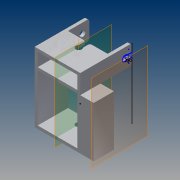
# Autodesk Inventor part: Box
Saved by Autodesk Inventor 2015 SP1 (Build 190203100, 203)
## iProperties
Created: 2015-04-28
Part Number: Box
Material: ABS Plastic
Document SubType Name: Modeling
Designer: Trevor
Density: 1.06 g/cm^3
Appearance: Smooth - White
Author: Trevor
Autodesk Inventor part; units mm, degrees
ref_plane "YZ Plane" through (0, 0, 0) normal (1, 0, 0) x (0, 1, 0)
ref_plane "XZ Plane" through (0, 0, 0) normal (0, 1, 0) x (-1, 0, 0)
ref_plane "XY Plane" through (0, 0, 0) normal (0, 0, 1) x (1, 0, 0)
sketch "Sketch1" plane through (0, 0, 0) normal (0, 0, 1) x (1, 0, 0)
  line L0 (-136.0917, 57.7981) -> (-136.0917, 38.4916) projected
  line L1 (-204.3542, 87.8916) -> (-204.3542, 49.7916) projected
  line L2 (-131.3292, 42.3074) -> (-204.3542, 42.3074)
  line L3 (-204.3542, 42.3074) -> (-204.3542, -69.3801)
  line L4 (-204.3542, -69.3801) -> (-131.3292, -69.3801)
  line L5 (-131.3292, -69.3801) -> (-131.3292, 42.3074)
  line L6 (-131.3292, 43.3824) -> (-131.3292, 52.9074) projected
  line L7 (-204.3542, 87.8916) -> (-204.3542, 49.7916) projected
  line L8 (-165.4906, 16.3449) -> (-168.0727, 16.3449)
  line L9 (-170.1927, 37.5449) -> (-167.6106, 37.5449)
  line L10 (-163.0792, 42.3074) -> (-172.6042, 42.3074) projected
  point P0 (0, 0)
  dimension "d1" = 4.7625
  dimension "d2" = 85.725
  dimension "d30" = 21.2
  constraints: 12 end point, 3 collinear, 2 parallel, 1 horizontal, 1 perpendicular
  measures "d1" distance between parallel lines of L2 L9
  measures "d2" distance between parallel lines of L4 L8
  measures "d30" distance between parallel lines of L8 L9
extrude "Extrusion1" add sketch "Sketch1" against normal blind 82.55
shell "Shell1" thickness 4.7625 removed faces 2 at (-180.0125, 5.0782, -82.55) at (-180.0125, 5.0782, 0)
sketch "Sketch2" plane through (0, 0, -82.55) normal (0, 0, -1) x (-1, 0, 0)
  line L0 (170.1927, 16.3449) -> (167.6106, 16.3449) projected
  line L1 (164.4741, 11.5824) -> (171.2093, 11.5824) projected
  line L2 (199.5917, 37.5449) -> (199.5917, -64.6176) projected
  line L3 (136.0917, -64.6176) -> (136.0917, 37.5449) projected
  line L4 (199.5917, -64.6176) -> (199.5917, 37.5449) projected
  line L5 (199.5917, 11.5824) -> (136.0917, 11.5824)
  line L6 (136.0917, 11.5824) -> (136.0917, 16.3449)
  line L7 (136.0917, 16.3449) -> (199.5917, 16.3449)
  line L8 (199.5917, 16.3449) -> (199.5917, 11.5824)
  point P0 (0, 0)
  constraints: 8 end point, 2 collinear, 2 parallel, 2 point on line, 1 horizontal, 1 perpendicular
extrude "Extrusion2" add sketch "Sketch2" against normal up to surface (82.55 mm away)
sketch "Sketch3" plane through (-204.3542, 42.3074, 0) normal (0, 1, 0) x (1, 0, 0)
  line L0 (73.025, 82.55) -> (0, 82.55) projected
  line L1 (36.5125, 82.55) -> (36.5125, 0)
  line L2 (0, 0) -> (73.025, 0) projected
  arc A0 (33.1449, 30.6087) -> (40.6772, 36.2864) centre (36.5125, 33.9763) ccw
  line L3 (73.025, 0) -> (0, 0) projected
  line L4 (33.1449, 30.6087) -> (39.8801, 30.6087)
  line L5 (39.8801, 30.6087) -> (39.8801, 37.3439)
  line L6 (39.8801, 37.3439) -> (33.1449, 37.3439)
  line L7 (33.1449, 37.3439) -> (33.1449, 30.6087)
  line L8 (33.1449, 30.6087) -> (39.8801, 37.3439) construction
  line L9 (39.8801, 30.6087) -> (33.1449, 37.3439) construction
  line L10 (39.8801, 37.3439) -> (39.8801, 39.3666)
  line L11 (33.1449, 37.3439) -> (33.1449, 39.3666)
  arc A1 (39.8801, 39.3666) -> (40.6772, 36.2864) centre (46.2301, 39.3666) ccw
  arc A2 (32.3478, 36.2864) -> (33.1449, 39.3666) centre (26.7949, 39.3666) ccw
  line L12 (68.2625, 82.55) -> (68.2625, 0) projected
  line L13 (4.7625, 0) -> (4.7625, 82.55) projected
  line L14 (4.7625, 82.55) -> (68.2625, 82.55)
  line L15 (68.2625, 82.55) -> (68.2625, 48.5832)
  line L16 (68.2625, 48.5832) -> (4.7625, 48.5832)
  line L17 (4.7625, 48.5832) -> (4.7625, 82.55)
  line L18 (33.1449, 39.3666) -> (33.1449, 82.55)
  arc A3 (32.3478, 36.2864) -> (33.1449, 30.6087) centre (36.5125, 33.9763) ccw
  line L19 (39.8801, 39.3666) -> (39.8801, 82.55)
  arc A4 (40.6772, 36.2864) -> (32.3478, 36.2864) centre (36.5125, 33.9763) ccw
  point P0 (204.3542, 0)
  dimension "d8" = 33.9763
  dimension "d9" = 6.7352
  dimension "d10" = 6.35
  dimension "d11" = 14.6069
  constraints: 30 end point, 14 point on circle, 7 perpendicular, 5 centre point, 4 midpoint, 4 parallel, 4 point on line, 3 symmetric about line, 3 tangent, 2 horizontal, 1 other
  measures "d8" distance from line of L3 A0.centre
  measures "d9" distance of L4.end L5.end
  measures "d10" radius of A1
  measures "d11" distance from line of A0.centre L16
extrude "Extrusion3" cut sketch "Sketch3" against normal through all contours L12 L16 L19 L0 | L19 L16 L1 L0 | L1 L16 L18 L0 | L19 L10 A4 L1 L16 | L18 L16 L13 L0 | L1 A4 L11 L18 L16 | A1 A4 L10 | A4 L6 L1 | L1 L6 A4 | A4 A0 L5 | L5 L4 L1 L6 | A0 L4 L1 | L1 L4 A0 | L11 A4 A2 | L1 L4 L7 L6 | L7 A3 A4
fillet "Fillet1" radius 3.175 6 edges at (-171.2093, 39.9261, -48.5832) (-164.4741, 39.9261, -48.5832) (-164.4741, 13.9636, -48.5832) (-171.2093, 13.9636, -48.5832) (-164.4741, -66.9989, -48.5832) (-171.2093, -66.9989, -48.5832)
sketch "Sketch4" plane through (-131.3292, -69.3801, 0) normal (1, 0, 0) x (0, 0, -1)
  point P0 (0, 69.3801)
sketch "Sketch5" plane through (-131.3292, -69.3801, 0) normal (1, 0, 0) x (0, 0, -1)
  line L0 (75.4488, 92.9574) -> (82.55, 92.9574)
  line L1 (75.4488, 99.6926) -> (77.4716, 99.6926)
  line L2 (76.8437, 96.325) -> (67.3187, 96.325)
  arc A0 (77.4716, 92.9574) -> (74.3914, 92.1603) centre (77.4716, 86.6074) ccw
  arc A1 (74.3914, 100.4897) -> (77.4716, 99.6926) centre (77.4716, 106.0426) ccw
  line L3 (82.55, 111.6875) -> (82.55, 0) projected
  circle A2 centre (72.0812, 96.325) radius 4.7625
  line L4 (77.4716, 99.6926) -> (82.55, 99.6926)
  arc A3 (74.3914, 100.4897) -> (74.3914, 92.1603) centre (72.0812, 96.325) ccw
  line L5 (82.55, 99.6926) -> (82.55, 92.9574)
  arc A4 (75.4488, 99.6926) -> (74.3914, 100.4897) centre (72.0812, 96.325) ccw
  arc A5 (74.3914, 92.1603) -> (75.4488, 99.6926) centre (72.0812, 96.325) ccw
  line L6 (75.4488, 99.6926) -> (68.7136, 99.6926)
  line L7 (68.7136, 92.9574) -> (75.4488, 92.9574)
  circle A6 centre (72.0812, 96.325) radius 4.7625
  point P0 (0, 69.3801)
  dimension "d15" = 6.35
  constraints: 15 point on circle, 14 end point, 6 centre point, 6 horizontal, 3 point on line, 2 coincident, 2 collinear, 2 symmetric about line, 1 horizontal alignment, 1 midpoint, 1 tangent, 10 other
  measures "d15" radius of A0
extrude "Extrusion4" cut sketch "Sketch5" against normal through all contours L7 A2 L2 | A2 L7 | L2 A2 L6 | L6 A2
extrude "Extrusion9" cut sketch "Sketch5" against normal up to surface (4.7625 mm away) contours A2 L1 L4 L3 L0 | L0 A0 A2 | A2 A1 L1
fillet "Fillet2" radius 3.175 2 edges at (-133.7104, 23.5773, -82.55) (-133.7104, 30.3125, -82.55)
sketch "Sketch8" plane through (-131.3292, -69.3801, 0) normal (1, 0, 0) x (0, 0, -1)
  arc A0 (62.5423, 84.4369) -> (84.9847, 88.2121) centre (72.0812, 96.325) ccw projected
  line L0 (48.5832, 85.725) -> (48.5832, 80.9625) projected
  line L1 (0, 0) -> (82.55, 0) projected
  line L2 (82.55, 111.6875) -> (82.55, 0) projected
  line L3 (82.55, 80.9625) -> (48.5832, 80.9625)
  line L4 (48.5832, 80.9625) -> (48.5832, 0)
  line L5 (48.5832, 0) -> (82.55, 0)
  line L6 (82.55, 0) -> (82.55, 80.9625)
  line L7 (0, 111.6875) -> (82.55, 111.6875) projected
  point P0 (0, 69.3801)
  point P1 (82.55, 92.1637)
  dimension "d38" = 30.725
  constraints: 8 end point, 2 parallel, 2 point on line, 1 collinear, 1 horizontal, 1 perpendicular
  measures "d38" distance between parallel lines of L7 L3
extrude "Extrusion6" cut sketch "Sketch8" against normal through all
fillet "Fillet3" radius 3.175 4 edges at (-201.9729, 11.5824, -82.55) (-201.9729, 42.3074, -82.55) (-133.7104, 42.3074, -82.55) (-133.7104, 11.5824, -82.55)
sketch "Sketch9" plane through (-131.3292, -69.3801, 0) normal (1, 0, 0) x (0, 0, -1)
  line L0 (45.4082, 80.9625) -> (48.5832, 80.9625) projected
  line L1 (45.4082, 80.9625) -> (39.3666, 80.9625) projected
  line L2 (39.3666, 80.9625) -> (36.2864, 80.9625) projected
  line L3 (36.2864, 80.9625) -> (36.2864, 80.9625) projected
  line L4 (36.2864, 80.9625) -> (39.3666, 80.9625) projected
  line L5 (39.3666, 80.9625) -> (45.4082, 80.9625) projected
  line L6 (48.5832, 80.9625) -> (45.4082, 80.9625) projected
  line L7 (0, 80.9625) -> (48.5832, 80.9625) projected
  line L8 (48.5832, 80.9625) -> (0, 80.9625) projected
  line L9 (48.5832, 80.9625) -> (32.3888, 80.9625)
  line L10 (32.3888, 80.9625) -> (32.3888, 0)
  line L11 (32.3888, 0) -> (48.5832, 0)
  line L12 (48.5832, 0) -> (48.5832, 80.9625)
  line L13 (33.9763, 134.025) -> (33.9763, -22.3375) projected
  dimension "d39" = 1.5875
  constraints: 8 end point, 2 parallel, 1 horizontal, 1 perpendicular
  measures "d39" distance between parallel lines of L13 L10
extrude "Extrusion7" cut sketch "Sketch9" against normal up to surface (4.7625 mm away)
ref_plane "Work Plane2" through (-167.8417, 42.3074, -33.9763) normal (-1, 0, 0) x (0, -1, 0)
sketch "Sketch10" plane through (-131.3292, -69.3801, 0) normal (1, 0, 0) x (0, 0, -1)
  line L0 (32.3888, 0) -> (32.3888, 80.9625)
  line L1 (0, 0) -> (32.3888, 0)
  line L2 (0, 0) -> (0, 111.6875)
  line L3 (32.3888, 80.9625) -> (0, 80.9625)
  line L4 (0, 80.9625) -> (0, 0)
  line L5 (0, 0) -> (32.3888, 0)
  line L6 (32.3888, 0) -> (32.3888, 80.9625)
  constraints: 14 end point, 2 parallel, 1 horizontal, 1 perpendicular
ref_plane "Work Plane1" through (-109.6917, 42.3074, -33.9763) normal (1, 0, 0) x (0, 1, 0)
extrude "Extrusion8" add sketch "Sketch10" along normal up to surface (21.6375 mm away)
sketch "Sketch11" plane through (-136.0917, -64.6176, -32.3888) normal (0, 0, -1) x (-1, 0, 0)
  line L0 (-26.4, 76.2) -> (5.35, 76.2)
  line L1 (5.35, 76.2) -> (5.35, 0)
  line L2 (5.35, 0) -> (-26.4, 0)
  line L3 (-26.4, 0) -> (-26.4, 76.2)
  line L4 (0, 0) -> (25.2074, 0) projected
  point P0 (-199.5917, 64.6176)
  point P1 (-20.05, 57.15)
  point P2 (-13.7, 19.05)
  dimension "d40" = 31.75
  dimension "d41" = 38.1
  dimension "d42" = 38.1
  dimension "d43" = 12.7
  dimension "d44" = 25.4
  constraints: 8 end point, 2 parallel, 1 collinear, 1 horizontal, 1 perpendicular
  measures "d40" distance between parallel lines of L3 L1
  measures "d41" diameter of point (-20.05, 57.15) L0
  measures "d42" diameter of point (-13.7, 19.05) L2
  measures "d43" diameter of point (-20.05, 57.15) L3
  measures "d44" diameter of point (-13.7, 19.05) L3
hole "Hole1" at (-116.0417, -7.4676, -32.3888) at (-122.3917, -45.5676, -32.3888) direction (0, 0, 1) diameter 2.81 depth 15
equation "\"d1\" = t"
equation "\"d30\" = w_gear"
equation "\"d5\" = t"
equation "\"d8\" = r_gear + t"
equation "\"d9\" = l_key"
equation "\"d11\" = 0.5 * r_gear"
equation "\"d38\" = w_gear + 2 * t"
equation "\"t\" = 4.7625"
equation "\"w_gear\" = 21.2"
equation "\"r_gear\" = 29.213787"
equation "\"l_key\" = 6.735192"
body "Solid1"
